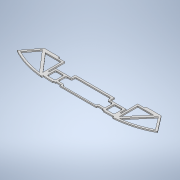
# Autodesk Inventor part: bulkhead_F1
Saved by Autodesk Inventor 2020.3 (Build 243373010, 373A)
## iProperties
Created: 2020-05-22
Part Number: bulkhead_F1
Material: Generic
Document SubType Name: Modeling
Designer: kardo
Density: 1 g/cm^3
Appearance: Default
Mass: 4.80884 g
Surface Area: 75.5406 cm^2
Volume: 4.80884 cm^3
Author: kardo
Autodesk Inventor part; units mm, degrees
ref_plane "YZ Plane" through (0, 0, 0) normal (1, 0, 0) x (0, 1, 0)
ref_plane "XZ Plane" through (0, 0, 0) normal (0, 1, 0) x (-1, 0, 0)
ref_plane "XY Plane" through (0, 0, 0) normal (0, 0, 1) x (1, 0, 0)
derived "base_sketch.ipt"
sketch "bulkhead_F1" plane through (0, 56.1, 0) normal (0, 1, 0) x (-1, 0, 0)
  line L0 (19.176, 46.818) -> (62.322, 46.818)
  line L1 (-34.5168, -2.4868) -> (-57.528, 27.54)
  line L2 (-11.5056, -2.4868) -> (-34.5168, -2.4868)
  line L3 (-11.5056, 0) -> (-11.5056, -2.4868)
  line L4 (0, 0) -> (-11.5056, 0)
  line L5 (62.322, 46.818) -> (62.322, 13.529)
  line L6 (28.764, 19.935) -> (28.764, 13.529)
  line L7 (-37.5231, 1.4361) -> (-11.5056, 1.4361)
  line L8 (-11.5056, 1.4361) -> (-11.5056, 3.9229)
  line L9 (-11.5056, 3.9229) -> (0, 3.9229)
  line L10 (0, 3.9229) -> (0, 21.6458)
  line L11 (0, 21.6458) -> (28.764, 21.6458)
  line L12 (28.764, 21.6458) -> (28.764, 14.7544)
  line L13 (28.764, 14.7544) -> (62.322, 14.7544)
  line L14 (62.322, 43.2359) -> (19.176, 43.2359)
  line L15 (-57.528, 27.54) -> (-37.5231, 1.4361)
  line L16 (0, 45.9) -> (0, 44.8052) construction
  line L17 (-19.176, 42.5952) -> (-19.176, 41.8654) construction
  line L18 (-38.352, 36.72) -> (-38.352, 36.3551) construction
  line L19 (0, 19.935) -> (0, 0)
  line L20 (0, 44.8052) -> (0, 42.3179)
  spline S0 degree 4 poles (-57.528, 27.54) (-46.0483, 34.2051) (-30.6129, 40.5281) (-11.2214, 45.0414) (8.3201, 46.818) (15.5662, 46.818) (19.176, 46.818) knots 0 0 0 0 0 0.630279 0.815816 1 1 1 1 1
  spline S1 degree 3 poles (-57.528, 27.54) (-39.1506, 37.8756) (-19.5945, 42.9173) (0, 44.8052) knots 0 0 0 0 1 1 1 1
  spline S2 degree 2 poles (0, 42.3179) (9.5715, 43.2359) (19.176, 43.2359) knots 0 0 0 1 1 1
  line L21 (0, 35.7) -> (-57.528, 27.54) construction
  line L22 (-11.5056, 1.4361) -> (0, 1.4361) construction
  line L23 (0, 1.4361) -> (0, 3.9229) construction
  point P0 (0, 14.7544)
  point P1 (0, 44.0613)
ref_plane "bulkhead_F1_plane" through (0, 56.1, 0) normal (0, 1, 0) x (-1, 0, 0)
sketch "Sketch2" plane through (0, 56.1, 0) normal (0, 1, 0) x (-1, 0, 0)
  spline S0 degree 2 poles (0, 42.3179) (9.5715, 43.2359) (19.176, 43.2359) knots 0 0 0 1 1 1 projected
  line L0 (62.322, 43.2359) -> (19.176, 43.2359) projected
  line L1 (62.322, 46.818) -> (62.322, 13.529) projected
  line L2 (28.764, 14.7544) -> (62.322, 14.7544) projected
  line L3 (28.764, 21.6458) -> (28.764, 14.7544) projected
  line L4 (0, 21.6458) -> (28.764, 21.6458) projected
  line L5 (0, 3.9229) -> (0, 21.6458) projected
  line L6 (-11.5056, 3.9229) -> (0, 3.9229) projected
  line L7 (-11.5056, 1.4361) -> (-11.5056, 3.9229) projected
  line L8 (-37.5231, 1.4361) -> (-11.5056, 1.4361) projected
  line L9 (-57.528, 27.54) -> (-37.5231, 1.4361) projected
  spline S1 degree 3 poles (-57.528, 27.54) (-39.1506, 37.8756) (-19.5945, 42.9173) (0, 44.8052) knots 0 0 0 0 1 1 1 1 projected
  line L10 (-53.0141, 26.5819) -> (-36.761, 5.3737)
  line L11 (-36.761, 5.3737) -> (-5.8311, 41.1224)
  line L12 (-30.1313, 6.9229) -> (-3, 38.2811)
  line L13 (-3, 38.2811) -> (-3, 6.9229)
  line L14 (-3, 6.9229) -> (-30.1313, 6.9229)
  line L15 (0, 21.6458) -> (0, 31.9819)
  line L16 (0, 31.9819) -> (2, 31.9819)
  line L17 (2, 31.9819) -> (2, 21.6458)
  line L18 (19.176, 37.3179) -> (19.176, 26.6458)
  line L19 (17.176, 24.6458) -> (7, 24.6458)
  line L20 (5, 26.6458) -> (5, 37.3179)
  line L21 (7, 39.3179) -> (17.176, 39.3179)
  line L22 (22.176, 35.8359) -> (22.176, 26.6458)
  line L23 (31.764, 21.6458) -> (31.764, 19.7544)
  line L24 (33.764, 17.7544) -> (62.322, 17.7544)
  line L25 (24.176, 37.8359) -> (31.176, 37.8359)
  spline S2 degree 2 poles (-53.0141, 26.5819) (-30.7214, 38.0667) (-5.8311, 41.1224) knots 0 0 0 1 1 1
  line L26 (-5.8311, 41.1224) -> (-6.2231, 44.0967) construction
  line L27 (-30.072, 35.9594) -> (-30.9423, 38.8304) construction
  line L28 (-53.0141, 26.5819) -> (-54.412, 29.2363) construction
  line L29 (-53.0141, 26.5819) -> (-30.072, 35.9594) construction
  line L30 (-30.072, 35.9594) -> (-5.8311, 41.1224) construction
  line L31 (-37.5231, 1.4361) -> (0, 44.8052) construction
  arc A0 (17.176, 24.6458) -> (19.176, 26.6458) centre (17.176, 26.6458) ccw
  arc A1 (5, 26.6458) -> (7, 24.6458) centre (7, 26.6458) ccw
  arc A2 (7, 39.3179) -> (5, 37.3179) centre (7, 37.3179) ccw
  arc A3 (19.176, 37.3179) -> (17.176, 39.3179) centre (17.176, 37.3179) ccw
  arc A4 (24.176, 37.8359) -> (22.176, 35.8359) centre (24.176, 35.8359) ccw
  arc A5 (31.764, 19.7544) -> (33.764, 17.7544) centre (33.764, 19.7544) ccw
  line L32 (62.322, 43.2359) -> (62.322, 14.7544)
  line L33 (0, 44.8052) -> (0, 42.3179) projected
  line L34 (0, 44.8052) -> (2, 44.8052)
  line L35 (2, 44.8052) -> (2, 42.4997)
  line L36 (0, 42.3179) -> (0, 31.9819) construction
  line L37 (35.2624, 41.2359) -> (62.322, 41.2359)
  line L38 (31.176, 37.8359) -> (35.2624, 41.2359) construction
  line L39 (35.2624, 41.2359) -> (34.0119, 41.2359) construction
  line L40 (34.0119, 41.2359) -> (33.4835, 40.1026) construction
  line L41 (33.4835, 40.1026) -> (32.955, 38.9692)
  line L42 (32.955, 38.9692) -> (32.4265, 37.8359) construction
  line L43 (32.4265, 37.8359) -> (31.176, 37.8359) construction
  line L44 (19.176, 43.2359) -> (19.176, 42.0359)
  line L45 (19.176, 42.0359) -> (22.176, 42.0359)
  line L46 (22.176, 42.0359) -> (22.176, 40.8359)
  line L47 (22.176, 40.8359) -> (31.176, 40.8359)
  line L48 (31.176, 40.8359) -> (31.176, 43.2359)
  line L49 (22.176, 42.0359) -> (25.176, 42.0359) construction
  line L50 (25.176, 42.0359) -> (25.176, 43.2359) construction
  spline S3 degree 3 poles (31.176, 37.8359) (31.9342, 37.8359) (32.6346, 38.2821) (32.955, 38.9692) knots 0 0 0 0 1 1 1 1
  spline S4 degree 3 poles (33.4835, 40.1026) (33.8039, 40.7897) (34.5043, 41.2359) (35.2624, 41.2359) knots 0 0 0 0 1 1 1 1
  spline S5 degree 3 poles (22.176, 26.6458) (22.176, 25.3818) (23.2185, 24.2966) (24.4815, 24.2458) knots 0 0 0 0 1 1 1 1
  spline S6 degree 3 poles (31.764, 21.6458) (31.764, 22.9098) (30.7215, 23.9951) (29.4585, 24.0458) knots 0 0 0 0 1 1 1 1
  line L51 (24.4815, 24.2458) -> (29.4585, 24.0458)
  line L52 (24.4815, 24.2458) -> (22.176, 24.3385) construction
  line L53 (22.176, 24.3385) -> (22.176, 26.6458) construction
  line L54 (29.4585, 24.0458) -> (31.764, 23.9532) construction
  line L55 (31.764, 23.9532) -> (31.764, 21.6458) construction
  line L56 (22.176, 26.6458) -> (31.764, 21.6458) construction
  point P0 (0, 0)
  point P1 (-57.528, 25.7972)
  point P2 (0, 44.0613)
  point P3 (33.2192, 39.5359)
  point P4 (26.97, 24.1458)
  dimension "d1" = 3
  dimension "d2" = 3
  dimension "d3" = 3
  dimension "d4" = 4
  dimension "d5" = 2
  dimension "d6" = 3
  dimension "d7" = 3
  dimension "d8" = 3
  dimension "d11" = 3
  dimension "d12" = 3
  dimension "d15" = 3
  dimension "d16" = 2
  dimension "d19" = 3
  dimension "d21" = 2
  dimension "d23" = 6
  dimension "d24" = 6
  dimension "d25" = 1.2
  dimension "d26" = 1.2
  dimension "d27" = 115
  dimension "d28" = 3
  dimension "d29" = 0.2
  dimension "d30" = 5
  constraints: 92 end point, 12 point on circle, 12 tangent, 11 parallel, 10 equal length, 10 vertical, 9 point on line, 7 collinear, 6 centre point, 6 horizontal, 6 perpendicular, 5 equal radius, 4 midpoint, 25 other
  measures "d1" distance between parallel lines of L6 L14
  measures "d2" distance between parallel lines of L5 L13
  measures "d4" distance between parallel lines of L12 L11
  measures "d5" distance between parallel lines of L17 L15
  measures "d6" distance between parallel lines of L20 L17
  measures "d7" distance from line of L33.end L21
  measures "d8" distance between parallel lines of L4 L19
  measures "d11" distance between parallel lines of L2 L24
  measures "d12" distance between parallel lines of L3 L23
  measures "d15" distance of L10.start L28.end
  measures "d16" radius of A0
  measures "d19" distance between parallel lines of L22 L18
  measures "d21" distance between parallel lines of L37 L0
  measures "d23" distance between parallel lines of L44 L50
  measures "d24" distance between parallel lines of L48 L50
  measures "d25" distance of L0.end L44.end
  measures "d26" distance of L45.end L46.end
  measures "d27" angle of L25 L41
  measures "d28" distance between parallel lines of L25 L47
  measures "d29" vertical distance of L51.start L51.end
  measures "d30" distance from line of L4 L22.end
extrude "Extrusion1" add sketch "Sketch2" along normal blind 2 contours L33 L34 L35 S0 | S0 L44 L45 L46 L47 L48 L0 L1 L37 S4 L41 S3 L25 A4 L22 S5 L51 S6 L23 A5 L24 L2 L3 L4 L17 L16 L15 L5 L6 L7 L8 L9 S1 L33
mirror "Mirror1" about plane through (-62.322, 56.1, 14.7544) normal (-1, 0, 0) of "Extrusion1"
equation "\"d5\" = stringer_thickness"
equation "\"d23\" = cowl_strip_width"
equation "\"d24\" = cowl_insulation_width"
equation "\"d25\" = decking_thickness"
equation "\"d26\" = decking_thickness"
equation "\"d17\" = bulkhead_thickness"
equation "\"stringer_thickness\" = 2"
equation "\"cowl_strip_width\" = 6"
equation "\"cowl_insulation_width\" = 6"
equation "\"decking_thickness\" = 1.2"
equation "\"bulkhead_thickness\" = 2"
body "Solid1"
